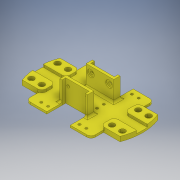
# Autodesk Inventor part: yellow_part-july21
Saved by Autodesk Inventor 2017 SP1 (Build 210196100, 196)
## iProperties
Created: 2016-07-25
Part Number: yellow_part-july21
Material: Verre
Document SubType Name: Modeling
Designer: tmonglon
Density: 2.18 g/cm^3
Appearance: Jaune canari
Mass: 28.4543 g
Surface Area: 129.801 cm^2
Volume: 13.0524 cm^3
Author: tmonglon
Autodesk Inventor part; units mm, degrees
(part 1 of 2)
ref_plane "YZ Plane" through (0, 0, 0) normal (1, 0, 0) x (0, 1, 0)
ref_plane "XZ Plane" through (0, 0, 0) normal (0, 1, 0) x (-1, 0, 0)
ref_plane "XY Plane" through (0, 0, 0) normal (0, 0, 1) x (1, 0, 0)
sketch "Esquisse1" plane through (0, 0, 0) normal (0, 0, 1) x (1, 0, 0)
  line L0 (-50, 42) -> (-50, 18)
  line L1 (-100, 30) -> (0, 30)
  line L2 (-61, 42) -> (-39, 42)
  line L3 (-77, 60) -> (-61.2, 60)
  line L4 (-38.8, 60) -> (-23, 60)
  line L5 (-81, 56) -> (-81, 47.873)
  line L6 (-19, 56) -> (-19, 47.873)
  line L7 (-81, 48) -> (-96.6476, 48)
  line L8 (-19, 48) -> (-3.3524, 48)
  line L9 (-96, 45) -> (-91, 45)
  line L10 (-91, 45) -> (-91, 40)
  line L11 (-91, 40) -> (-96, 40)
  line L12 (-96, 40) -> (-96, 45)
  line L13 (-91, 44) -> (-94, 44)
  line L14 (-94, 44) -> (-94, 41)
  line L15 (-94, 41) -> (-91, 41)
  line L16 (-91, 41) -> (-91, 44)
  line L17 (-86, 45) -> (-81, 45)
  line L18 (-81, 45) -> (-81, 40)
  line L19 (-81, 40) -> (-86, 40)
  line L20 (-86, 40) -> (-86, 45)
  line L21 (-4, 45) -> (-9, 45)
  line L22 (-9, 45) -> (-9, 40)
  line L23 (-9, 40) -> (-4, 40)
  line L24 (-4, 40) -> (-4, 45)
  line L25 (-9, 44) -> (-6, 44)
  line L26 (-6, 44) -> (-6, 41)
  line L27 (-6, 41) -> (-9, 41)
  line L28 (-9, 41) -> (-9, 44)
  line L29 (-14, 45) -> (-19, 45)
  line L30 (-19, 45) -> (-19, 40)
  line L31 (-19, 40) -> (-14, 40)
  line L32 (-14, 40) -> (-14, 45)
  line L33 (-96, 15) -> (-91, 15)
  line L34 (-91, 15) -> (-91, 20)
  line L35 (-91, 20) -> (-96, 20)
  line L36 (-96, 20) -> (-96, 15)
  line L37 (-91, 16) -> (-94, 16)
  line L38 (-94, 16) -> (-94, 19)
  line L39 (-94, 19) -> (-91, 19)
  line L40 (-91, 19) -> (-91, 16)
  line L41 (-86, 15) -> (-81, 15)
  line L42 (-81, 15) -> (-81, 20)
  line L43 (-81, 20) -> (-86, 20)
  line L44 (-86, 20) -> (-86, 15)
  line L45 (-19, 15) -> (-19, 20)
  line L46 (-14, 15) -> (-19, 15)
  line L47 (-14, 20) -> (-14, 15)
  line L48 (-19, 20) -> (-14, 20)
  line L49 (-9, 16) -> (-6, 16)
  line L50 (-6, 19) -> (-9, 19)
  line L51 (-6, 16) -> (-6, 19)
  line L52 (-4, 15) -> (-9, 15)
  line L53 (-4, 20) -> (-4, 15)
  line L54 (-9, 20) -> (-4, 20)
  line L55 (-9, 19) -> (-9, 16)
  line L56 (-9, 15) -> (-9, 20)
  line L57 (-61, 18) -> (-39, 18)
  line L58 (-77, 0) -> (-61.2, 0)
  line L59 (-38.8, 0) -> (-23, 0)
  line L60 (-81, 4) -> (-81, 12.127)
  line L61 (-19, 4) -> (-19, 12.127)
  line L62 (-81, 12) -> (-96.6476, 12)
  line L63 (-19, 12) -> (-3.3524, 12)
  arc A0 (-96.6476, 48) -> (-96.6476, 12) centre (-50, 30) ccw
  arc A1 (-3.3524, 12) -> (-3.3524, 48) centre (-50, 30) ccw
  arc A2 (-96.6476, 48) -> (-96.6476, 12) centre (-50, 30) ccw
  arc A3 (-3.3524, 12) -> (-3.3524, 48) centre (-50, 30) ccw
  line L64 (-23, 0) -> (-38.8, 0)
  line L65 (-61.2, 0) -> (-77, 0)
  line L66 (-78, 44) -> (-78, 39)
  line L67 (-82, 35) -> (-98.5, 35)
  line L68 (-81, 48) -> (-82, 48)
  arc A4 (-82, 35) -> (-78, 39) centre (-82, 39) ccw
  arc A5 (-78, 44) -> (-82, 48) centre (-82, 44) ccw
  arc A6 (-99.707, 35.4053) -> (-98.5, 35) centre (-98.5, 37) ccw
  line L69 (-22, 44) -> (-22, 39)
  line L70 (-18, 35) -> (-1.5, 35)
  arc A7 (-22, 39) -> (-18, 35) centre (-18, 39) ccw
  arc A8 (-18, 48) -> (-22, 44) centre (-18, 44) ccw
  arc A9 (-1.5, 35) -> (-0.293, 35.4053) centre (-1.5, 37) ccw
  line L71 (-78, 16) -> (-78, 21)
  line L72 (-82, 25) -> (-98.5, 25)
  arc A10 (-78, 21) -> (-82, 25) centre (-82, 21) ccw
  arc A11 (-82, 12) -> (-78, 16) centre (-82, 16) ccw
  arc A12 (-98.5, 25) -> (-99.707, 24.5947) centre (-98.5, 23) ccw
  arc A13 (-22, 16) -> (-18, 12) centre (-18, 16) ccw
  line L73 (-22, 16) -> (-22, 21)
  arc A14 (-18, 25) -> (-22, 21) centre (-18, 21) ccw
  line L74 (-18, 25) -> (-1.5, 25)
  arc A15 (-0.293, 24.5947) -> (-1.5, 25) centre (-1.5, 23) ccw
  arc A16 (-77, 60) -> (-81, 56) centre (-77, 56) ccw
  arc A17 (-19, 56) -> (-23, 60) centre (-23, 56) ccw
  arc A18 (-81, 4) -> (-77, 0) centre (-77, 4) ccw
  arc A19 (-23, 0) -> (-19, 4) centre (-23, 4) ccw
  circle A20 centre (-60, 26.75) radius 1
  circle A21 centre (-40, 26.75) radius 1
  circle A22 centre (-40, 33.25) radius 1
  circle A23 centre (-60, 33.25) radius 1
  line L75 (-61, 18) -> (-61.2, 18)
  line L76 (-61.2, 18) -> (-61.2, 0)
  line L77 (-39, 18) -> (-38.8, 18)
  line L78 (-38.8, 18) -> (-38.8, 0)
  line L79 (-61, 42) -> (-61.2, 42)
  line L80 (-61.2, 42) -> (-61.2, 60)
  line L81 (-39, 42) -> (-38.8, 42)
  line L82 (-38.8, 42) -> (-38.8, 60)
  circle A24 centre (-71.5, 55) radius 1
  circle A25 centre (-65, 55) radius 1
  circle A26 centre (-28.5, 55) radius 1
  circle A27 centre (-35, 55) radius 1
  circle A28 centre (-71.5, 5) radius 1
  circle A29 centre (-65, 5) radius 1
  circle A30 centre (-35, 5) radius 1
  circle A31 centre (-28.5, 5) radius 1
  point P0 (0, 0)
  point P1 (-100, 48)
  point P2 (0, 48)
  point P3 (-81, 60)
  point P4 (-19, 60)
  point P5 (-81, 0)
  point P6 (-19, 0)
  dimension "d4" = 22
  dimension "d9" = 5
  dimension "d10" = 5
  dimension "d11" = 3
  dimension "d12" = 3
  dimension "d13" = 1
  dimension "d14" = 10
  dimension "d16" = 5
  dimension "d17" = 5
  dimension "d18" = 5
  dimension "d19" = 22
  dimension "d20" = 13
  dimension "d21" = 4
  dimension "d23" = 4
  dimension "d24" = 1.5
  dimension "d25" = 4
  dimension "d26" = 2
  dimension "d27" = 2
  dimension "d28" = 2
  dimension "d29" = 2
  dimension "d30" = 10
  dimension "d31" = 10
  dimension "d32" = 10
  dimension "d33" = 10
  dimension "d34" = 3.25
  dimension "d35" = 3.25
  dimension "d36" = 3.25
  dimension "d37" = 3.25
  dimension "d42" = 22.4
  dimension "d43" = 22.4
  dimension "d44" = 2
  dimension "d45" = 2
  dimension "d46" = 6.5
  dimension "d47" = 28.5
  dimension "d48" = 5
  constraints: 166 end point, 75 symmetric about line, 50 point on circle, 32 centre point, 24 point on line, 13 tangent, 11 horizontal, 10 parallel, 8 perpendicular, 4 equal radius, 3 midpoint, 2 vertical, 15 other
  measures "d4" distance of L2.start L2.end
  measures "d9" distance of L10.end L11.end
  measures "d10" distance of L9.end L10.end
  measures "d11" distance of L13.start L13.end
  measures "d12" distance of L13.end L14.end
  measures "d13" distance between parallel lines of L9 L13
  measures "d14" distance between parallel lines of L1 L11
  measures "d16" distance of L17.start L17.end
  measures "d17" distance of L17.end L18.end
  measures "d18" distance between parallel lines of L20 L16
  measures "d19" distance from line of L66 L1.start
  measures "d20" distance between parallel lines of L67 L7
  measures "d21" radius of A4
  measures "d23" diameter of A6
  measures "d24" horizontal distance of L1.start A6.centre
  measures "d25" radius of A16
  measures "d26" diameter of A20
  measures "d27" diameter of A21
  measures "d28" diameter of A22
  measures "d29" diameter of A23
  measures "d30" distance from line of L0 A23.centre
  measures "d31" distance from line of L0 A22.centre
  measures "d32" distance from line of L0 A20.centre
  measures "d33" distance from line of A21.centre L0
  measures "d34" distance from line of L1 A23.centre
  measures "d35" distance from line of L1 A20.centre
  measures "d36" distance from line of L1 A21.centre
  measures "d37" distance from line of L1 A22.centre
  measures "d42" distance between parallel lines of L82 L80
  measures "d43" distance between parallel lines of L78 L76
  measures "d44" diameter of A24
  measures "d45" diameter of A25
  measures "d46" distance of A25.centre A24.centre
  measures "d47" horizontal distance of L1.start A24.centre
  measures "d48" distance from line of L3 A24.centre
extrude "Extrusion1" add sketch "Esquisse1" against normal blind 2 contours L2 L81 L82 L4 A17 L6 A8 L69 A7 L70 A9 A1 L1 L0 | L0 L1 A0 A6 L67 A4 L66 A5 L5 A16 L3 L80 L79 L2 | L1 A1 A15 L74 A14 L73 A13 L61 A19 L59 L78 L77 L57 L0 | L0 L57 L75 L76 L58 A18 L60 A11 L71 A10 L72 A12 A0 L1 | A0 L7 A5 L66 A4 L67 A6 | A12 L72 A10 L71 A11 L62 A0 | A1 L63 A13 L73 A14 L74 A15 | A9 L70 A7 L69 A8 L8 A1 | L7 L5 A5 | A11 L60 L62 | L63 L61 A13 | A8 L6 L8 | L9 L10 L13 L14 L15 L11 L12 | L24 L23 L22 L27 L26 L25 L21 | L36 L35 L34 L39 L38 L37 L33 | L49 L51 L50 L56 L54 L53 L52
extrude "Extrusion3" add sketch "Esquisse1" along normal blind 2.5 contours A0 L7 A5 L66 A4 L67 A6 | L9 L10 L13 L14 L15 L11 L12
extrude "Extrusion4" add sketch "Esquisse1" along normal blind 2.5 contours A1 L63 A13 L73 A14 L74 A15 | L49 L51 L50 L56 L54 L53 L52
sketch "Esquisse4" plane through (0, 0, 0) normal (0, 0, 1) x (1, 0, 0)
  line L0 (-91, 44) -> (-91, 41) projected
  line L1 (-91, 41) -> (-94, 41) projected
  line L2 (-94, 41) -> (-94, 44) projected
  line L3 (-94, 44) -> (-91, 44) projected
  arc A0 (-78, 44) -> (-82, 48) centre (-82, 44) ccw projected
  line L4 (-82, 48) -> (-96.6476, 48) projected
  arc A1 (-96.6476, 48) -> (-99.707, 35.4053) centre (-50, 30) ccw projected
  arc A2 (-99.707, 35.4053) -> (-98.5, 35) centre (-98.5, 37) ccw projected
  line L5 (-98.5, 35) -> (-82, 35) projected
  arc A3 (-82, 35) -> (-78, 39) centre (-82, 39) ccw projected
  line L6 (-78, 39) -> (-78, 44) projected
  line L7 (-81, 45) -> (-81, 40) projected
  line L8 (-81, 40) -> (-86, 40) projected
  line L9 (-86, 40) -> (-86, 45) projected
  line L10 (-86, 45) -> (-81, 45) projected
  line L11 (-9, 16) -> (-9, 19) projected
  line L12 (-9, 19) -> (-6, 19) projected
  line L13 (-6, 19) -> (-6, 16) projected
  line L14 (-6, 16) -> (-9, 16) projected
  line L15 (-19, 15) -> (-19, 20) projected
  line L16 (-19, 20) -> (-14, 20) projected
  line L17 (-14, 20) -> (-14, 15) projected
  line L18 (-14, 15) -> (-19, 15) projected
  arc A4 (-3.3524, 12) -> (-0.293, 24.5947) centre (-50, 30) ccw projected
  arc A5 (-0.293, 24.5947) -> (-1.5, 25) centre (-1.5, 23) ccw projected
  line L19 (-1.5, 25) -> (-18, 25) projected
  arc A6 (-18, 25) -> (-22, 21) centre (-18, 21) ccw projected
  line L20 (-22, 21) -> (-22, 16) projected
  arc A7 (-22, 16) -> (-18, 12) centre (-18, 16) ccw projected
  line L21 (-18, 12) -> (-3.3524, 12) projected
  line L22 (-50, 30) -> (-66.4619, 30)
  line L23 (-91, 16) -> (-91, 19)
  line L24 (-91, 19) -> (-94, 19)
  line L25 (-94, 19) -> (-94, 16)
  line L26 (-94, 16) -> (-91, 16)
  arc A8 (-82, 12) -> (-78, 16) centre (-82, 16) ccw
  line L27 (-82, 12) -> (-96.6476, 12)
  arc A9 (-99.707, 24.5947) -> (-96.6476, 12) centre (-50, 30) ccw
  arc A10 (-98.5, 25) -> (-99.707, 24.5947) centre (-98.5, 23) ccw
  line L28 (-98.5, 25) -> (-82, 25)
  arc A11 (-78, 21) -> (-82, 25) centre (-82, 21) ccw
  line L29 (-78, 21) -> (-78, 16)
  line L30 (-81, 15) -> (-81, 20)
  line L31 (-81, 20) -> (-86, 20)
  line L32 (-86, 20) -> (-86, 15)
  line L33 (-86, 15) -> (-81, 15)
  line L34 (-9, 44) -> (-9, 41)
  line L35 (-9, 41) -> (-6, 41)
  line L36 (-6, 41) -> (-6, 44)
  line L37 (-6, 44) -> (-9, 44)
  line L38 (-19, 45) -> (-19, 40)
  line L39 (-19, 40) -> (-14, 40)
  line L40 (-14, 40) -> (-14, 45)
  line L41 (-14, 45) -> (-19, 45)
  arc A12 (-0.293, 35.4053) -> (-3.3524, 48) centre (-50, 30) ccw
  arc A13 (-1.5, 35) -> (-0.293, 35.4053) centre (-1.5, 37) ccw
  line L42 (-1.5, 35) -> (-18, 35)
  arc A14 (-22, 39) -> (-18, 35) centre (-18, 39) ccw
  line L43 (-22, 39) -> (-22, 44)
  arc A15 (-18, 48) -> (-22, 44) centre (-18, 44) ccw
  line L44 (-18, 48) -> (-3.3524, 48)
  point P0 (0, 0)
  constraints: 46 end point, 36 symmetric about line, 16 point on circle, 8 centre point, 1 horizontal, 8 other
extrude "Extrusion5" add sketch "Esquisse4" along normal blind 2.5 contours L27 A9 A10 L28 A11 L29 A8 | A13 L42 A14 L43 A15 L44 A12
sketch "Esquisse6" plane through (0, 0, 2.5) normal (0, 0, 1) x (1, 0, 0)
  arc A0 (-98.5, 25) -> (-99.707, 24.5947) centre (-98.5, 23) ccw projected
  line L0 (-98.5, 25) -> (-82, 25) projected
  arc A1 (-78, 21) -> (-82, 25) centre (-82, 21) ccw projected
  line L1 (-78, 21) -> (-78, 16) projected
  arc A2 (-82, 12) -> (-78, 16) centre (-82, 16) ccw projected
  line L2 (-82, 12) -> (-96.6476, 12) projected
  arc A3 (-99.707, 24.5947) -> (-96.6476, 12) centre (-50, 30) ccw projected
  arc A4 (-1.5, 35) -> (-0.293, 35.4053) centre (-1.5, 37) ccw projected
  line L3 (-1.5, 35) -> (-18, 35) projected
  arc A5 (-22, 39) -> (-18, 35) centre (-18, 39) ccw projected
  line L4 (-22, 39) -> (-22, 44) projected
  arc A6 (-18, 48) -> (-22, 44) centre (-18, 44) ccw projected
  line L5 (-18, 48) -> (-3.3524, 48) projected
  arc A7 (-0.293, 35.4053) -> (-3.3524, 48) centre (-50, 30) ccw projected
  arc A8 (-22, 16) -> (-18, 12) centre (-18, 16) ccw projected
  line L6 (-22, 16) -> (-22, 21) projected
  arc A9 (-18, 25) -> (-22, 21) centre (-18, 21) ccw projected
  line L7 (-18, 25) -> (-1.5, 25) projected
  arc A10 (-0.293, 24.5947) -> (-1.5, 25) centre (-1.5, 23) ccw projected
  arc A11 (-3.3524, 12) -> (-0.293, 24.5947) centre (-50, 30) ccw projected
  line L8 (-3.3524, 12) -> (-18, 12) projected
  arc A12 (-99.707, 35.4053) -> (-98.5, 35) centre (-98.5, 37) ccw projected
  arc A13 (-96.6476, 48) -> (-99.707, 35.4053) centre (-50, 30) ccw projected
  line L9 (-96.6476, 48) -> (-82, 48) projected
  arc A14 (-78, 44) -> (-82, 48) centre (-82, 44) ccw projected
  line L10 (-78, 44) -> (-78, 39) projected
  arc A15 (-82, 35) -> (-78, 39) centre (-82, 39) ccw projected
  line L11 (-82, 35) -> (-98.5, 35) projected
  line L12 (-14, 15) -> (-14, 20) projected
  line L13 (-14, 20) -> (-19, 20) projected
  line L14 (-19, 20) -> (-19, 15) projected
  line L15 (-19, 15) -> (-14, 15) projected
  line L16 (-86, 45) -> (-86, 40) projected
  line L17 (-86, 40) -> (-81, 40) projected
  line L18 (-81, 40) -> (-81, 45) projected
  line L19 (-81, 45) -> (-86, 45) projected
  line L20 (-81, 20) -> (-86, 20) projected
  line L21 (-86, 20) -> (-86, 15) projected
  line L22 (-86, 15) -> (-81, 15) projected
  line L23 (-81, 15) -> (-81, 20) projected
  line L24 (-9, 41) -> (-6, 41) projected
  line L25 (-6, 41) -> (-6, 44) projected
  line L26 (-6, 44) -> (-9, 44) projected
  line L27 (-9, 44) -> (-9, 41) projected
  line L28 (-19, 45) -> (-19, 40) projected
  line L29 (-19, 40) -> (-14, 40) projected
  line L30 (-14, 40) -> (-14, 45) projected
  line L31 (-14, 45) -> (-19, 45) projected
  line L32 (-94, 44) -> (-94, 41) projected
  line L33 (-94, 41) -> (-91, 41) projected
  line L34 (-91, 41) -> (-91, 44) projected
  line L35 (-91, 44) -> (-94, 44) projected
  line L36 (-6, 16) -> (-6, 19) projected
  line L37 (-6, 19) -> (-9, 19) projected
  line L38 (-9, 19) -> (-9, 16) projected
  line L39 (-9, 16) -> (-6, 16) projected
  line L40 (-91, 19) -> (-94, 19) projected
  line L41 (-94, 19) -> (-94, 16) projected
  line L42 (-94, 16) -> (-91, 16) projected
  line L43 (-91, 16) -> (-91, 19) projected
  line L44 (-91, 45) -> (-96, 45)
  line L45 (-96, 45) -> (-96, 40)
  line L46 (-96, 40) -> (-91, 40)
  line L47 (-91, 40) -> (-91, 45)
  line L48 (-91, 44) -> (-91, 41) projected
  line L49 (-91, 20) -> (-96, 20)
  line L50 (-96, 20) -> (-96, 15)
  line L51 (-96, 15) -> (-91, 15)
  line L52 (-91, 15) -> (-91, 20)
  line L53 (-50, 30) -> (-50, 35)
  line L54 (-6, 44) -> (-6, 41)
  line L55 (-6, 41) -> (-9, 41)
  line L56 (-9, 41) -> (-9, 44)
  line L57 (-9, 44) -> (-6, 44)
  line L58 (-9, 19) -> (-6, 19)
  line L59 (-6, 19) -> (-6, 16)
  line L60 (-6, 16) -> (-9, 16)
  line L61 (-9, 16) -> (-9, 19)
  line L62 (-9, 45) -> (-4, 45)
  line L63 (-4, 45) -> (-4, 40)
  line L64 (-4, 40) -> (-9, 40)
  line L65 (-9, 40) -> (-9, 45)
  line L66 (-9, 44) -> (-9, 41)
  line L67 (-9, 20) -> (-4, 20)
  line L68 (-4, 20) -> (-4, 15)
  line L69 (-4, 15) -> (-9, 15)
  line L70 (-9, 15) -> (-9, 20)
  point P0 (0, 0)
  dimension "d59" = 5
  dimension "d60" = 5
  dimension "d61" = 1
  dimension "d62" = 5
  dimension "d63" = 5
  dimension "d64" = 1
  constraints: 52 end point, 8 symmetric about line, 4 parallel, 2 horizontal, 2 perpendicular, 1 collinear, 1 vertical
  measures "d59" distance of L44.end L45.end
  measures "d60" distance of L45.end L46.end
  measures "d61" distance between parallel lines of L46 L33
  measures "d62" distance of L49.end L50.end
  measures "d63" distance of L49.start L49.end
  measures "d64" distance between parallel lines of L51 L42
extrude "Extrusion6" cut sketch "Esquisse6" against normal blind 3 contours L27 L26 L25 L24 | L24 L25 L26 L65 L62 L63 L64 | L35 L34 L33 L32 | L32 L33 L47 L46 L45 L44 L35 | L36 L37 L70 L67 L68 L69 L39 | L43 L42 L41 L40 | L40 L41 L42 L52 L51 L50 L49
sketch "Esquisse7" plane through (0, 0, -2) normal (0, 0, -1) x (-1, 0, 0)
  line L0 (91, 44) -> (94, 44) projected
  line L1 (94, 44) -> (94, 41) projected
  line L2 (94, 41) -> (91, 41) projected
  line L3 (91, 41) -> (91, 44) projected
  line L4 (86, 45) -> (86, 40) projected
  line L5 (86, 40) -> (81, 40) projected
  line L6 (81, 40) -> (81, 45) projected
  line L7 (81, 45) -> (86, 45) projected
  line L8 (91, 19) -> (94, 19) projected
  line L9 (94, 19) -> (94, 16) projected
  line L10 (94, 16) -> (91, 16) projected
  line L11 (91, 16) -> (91, 19) projected
  line L12 (81, 20) -> (86, 20) projected
  line L13 (86, 20) -> (86, 15) projected
  line L14 (86, 15) -> (81, 15) projected
  line L15 (81, 15) -> (81, 20) projected
  circle A0 centre (65, 5) radius 1 projected
  circle A1 centre (71.5, 5) radius 1 projected
  circle A2 centre (60, 26.75) radius 1 projected
  arc A3 (96.6476, 12) -> (96.6476, 48) centre (50, 30) ccw projected
  line L16 (96.6476, 48) -> (81, 48) projected
  line L17 (81, 48) -> (81, 56) projected
  arc A4 (81, 56) -> (77, 60) centre (77, 56) ccw projected
  line L18 (77, 60) -> (61.2, 60) projected
  line L19 (61.2, 60) -> (61.2, 42) projected
  line L20 (61.2, 42) -> (38.8, 42) projected
  line L21 (38.8, 42) -> (38.8, 60) projected
  line L22 (38.8, 60) -> (23, 60) projected
  arc A5 (23, 60) -> (19, 56) centre (23, 56) ccw projected
  line L23 (19, 56) -> (19, 48) projected
  line L24 (19, 48) -> (3.3524, 48) projected
  arc A6 (3.3524, 48) -> (3.3524, 12) centre (50, 30) ccw projected
  line L25 (3.3524, 12) -> (19, 12) projected
  line L26 (19, 12) -> (19, 4) projected
  arc A7 (19, 4) -> (23, 0) centre (23, 4) ccw projected
  line L27 (23, 0) -> (38.8, 0) projected
  line L28 (38.8, 0) -> (38.8, 18) projected
  line L29 (38.8, 18) -> (61.2, 18) projected
  line L30 (61.2, 18) -> (61.2, 0) projected
  line L31 (61.2, 0) -> (77, 0) projected
  arc A8 (77, 0) -> (81, 4) centre (77, 4) ccw projected
  line L32 (81, 4) -> (81, 12) projected
  line L33 (81, 12) -> (96.6476, 12) projected
  circle A9 centre (40, 33.25) radius 1 projected
  circle A10 centre (35, 55) radius 1 projected
  circle A11 centre (28.5, 55) radius 1 projected
  line L34 (19, 45) -> (19, 40) projected
  line L35 (19, 40) -> (14, 40) projected
  line L36 (14, 40) -> (14, 45) projected
  line L37 (14, 45) -> (19, 45) projected
  line L38 (9, 41) -> (6, 41) projected
  line L39 (6, 41) -> (6, 44) projected
  line L40 (6, 44) -> (9, 44) projected
  line L41 (9, 44) -> (9, 41) projected
  line L42 (14, 15) -> (14, 20) projected
  line L43 (14, 20) -> (19, 20) projected
  line L44 (19, 20) -> (19, 15) projected
  line L45 (19, 15) -> (14, 15) projected
  circle A12 centre (35, 5) radius 1 projected
  circle A13 centre (28.5, 5) radius 1 projected
  circle A14 centre (40, 26.75) radius 1 projected
  circle A15 centre (65, 55) radius 1 projected
  circle A16 centre (71.5, 55) radius 1 projected
  circle A17 centre (60, 33.25) radius 1 projected
  line L46 (9, 16) -> (6, 16) projected
  line L47 (6, 16) -> (6, 19) projected
  line L48 (6, 19) -> (9, 19) projected
  line L49 (9, 19) -> (9, 16) projected
  line L50 (61.2, 18) -> (38.8, 18)
  line L51 (38, 20.5) -> (62, 20.5)
  line L52 (61.2, 42) -> (38.8, 42)
  line L53 (38, 39.5) -> (62, 39.5)
  line L54 (61.2, 42) -> (38.8, 42) projected
  line L55 (38.8, 20.5) -> (36.8, 20.5)
  line L56 (36.8, 20.5) -> (36.8, 14.5)
  line L57 (36.8, 14.5) -> (38.8, 14.5)
  line L58 (38.8, 14.5) -> (38.8, 18)
  line L59 (38.8, 0) -> (38.8, 18) projected
  line L60 (38.8, 39.5) -> (36.8, 39.5)
  line L61 (36.8, 39.5) -> (36.8, 45.5)
  line L62 (36.8, 45.5) -> (38.8, 45.5)
  line L63 (38.8, 45.5) -> (38.8, 42)
  line L64 (61.1821, 39.5) -> (63.1821, 39.5)
  line L65 (63.1821, 39.5) -> (63.1821, 45.5)
  line L66 (63.1821, 45.5) -> (61.1821, 45.5)
  line L67 (61.1821, 45.5) -> (61.1821, 42)
  line L68 (61.1821, 20.5) -> (63.1821, 20.5)
  line L69 (63.1821, 20.5) -> (63.1821, 14.5)
  line L70 (63.1821, 14.5) -> (61.1821, 14.5)
  line L71 (61.1821, 14.5) -> (61.1821, 18)
  point P0 (0, 0)
  dimension "d70" = 22.4
  dimension "d72" = 6
  dimension "d73" = 2
  dimension "d74" = 2
  dimension "d75" = 6
  dimension "d76" = 2
  dimension "d77" = 6
  dimension "d78" = 2
  constraints: 40 end point, 13 point on line, 10 parallel, 6 horizontal, 4 perpendicular, 2 collinear
  measures "d70" distance between parallel lines of L30 L28
  measures "d72" distance of L55.end L56.end
  measures "d73" distance of L56.end L57.end
  measures "d74" distance of L61.end L62.end
  measures "d75" distance of L60.end L61.end
  measures "d76" distance of L65.end L66.end
  measures "d77" distance of L68.end L69.end
  measures "d78" distance of L69.end L70.end
extrude "Extrusion7" add sketch "Esquisse7" against normal blind 21 contours L70 L71 L29 L30 | L30 L29 L28 L57 L56 L55 L51 L68 L69 L70 | L66 L65 L64 L53 L60 L61 L62 L21 L20 L19 | L19 L20 L67 L66
sketch "Esquisse8" plane through (-61.1821, 18, -2) normal (0, -1, 0) x (1, 0, 0)
  line L0 (0, 21) -> (0, 0) projected
  line L1 (22.3821, 0) -> (0, 0) projected
  line L2 (22.3821, 0) -> (22.3821, 21) projected
  line L3 (0, 21) -> (22.3821, 21) projected
  line L4 (-2, 21) -> (24.3821, 21) projected
  line L5 (11.1911, 21) -> (11.1911, 2)
  line L6 (-2, 2) -> (24.3821, 2) projected
  circle A0 centre (2.4411, 15.2) radius 1.25
  circle A1 centre (19.9411, 15.2) radius 1.25
  point P0 (61.1821, 2)
  dimension "d81" = 2.5
  dimension "d82" = 5.8
  dimension "d83" = 8.75
  constraints: 2 centre point, 2 end point, 2 midpoint, 1 symmetric about line, 1 other
  measures "d81" diameter of A0
  measures "d82" distance from line of L3 A0.centre
  measures "d83" distance from line of L5 A0.centre
extrude "Extrusion8" cut sketch "Esquisse8" against normal through all contours A0 | A1
hole "Perçage1" at (-58.7411, 39.5, 13.2) direction (0, 1, 0) diameter 6.6 depth 1
hole "Perçage2" at (-41.2411, 39.5, 13.2) direction (0, 1, 0) diameter 6.6 depth 1
hole "Perçage3" at (-41.2411, 20.5, 13.2) direction (0, -1, 0) diameter 6.6 depth 1
hole "Perçage4" at (-58.7411, 20.5, 13.2) direction (0, -1, 0) diameter 6.6 depth 1
fillet "Congé1" radius 2 2 edges at (-49.9911, 20.5, 0) (-49.9911, 39.5, 0)
fillet "Congé2" radius 2 8 edges at (-36.8, 21.5, 0) (-36.8, 17.5, 0) (-36.8, 42.5, 0) (-36.8, 38.5, 0) (-63.1821, 21.5, 0) (-63.1821, 17.5, 0) (-63.1821, 42.5, 0) (-63.1821, 38.5, 0)
fillet "Congé3" radius 2 8 edges at (-35.8, 14.5, 0) (-37.8, 14.5, 0) (-64.1821, 14.5, 0) (-62.1911, 14.5, 0) (-62.1911, 45.5, 0) (-64.1821, 45.5, 0) (-37.8, 45.5, 0) (-35.8, 45.5, 0)
sketch "Esquisse9" plane through (0, 0, -2) normal (0, 0, -1) x (-1, 0, 0)
  line L0 (20.3471, 14.8582) -> (37.5767, 14.8582) construction
  line L1 (37.5767, 14.8582) -> (37.5767, 7.8153) construction
  line L2 (37.5767, 7.8153) -> (20.3471, 7.8153) construction
  line L3 (20.3471, 7.8153) -> (20.3471, 14.8582) construction
  line L4 (66.5479, 9.4629) -> (66.5479, 31.182) construction
  line L5 (66.5479, 31.182) -> (77.9246, 31.182) construction
  line L6 (77.9246, 31.182) -> (77.9246, 9.4629) construction
  line L7 (77.9246, 9.4629) -> (66.5479, 9.4629) construction
  line L8 (25.3892, 14.7346) -> (23.2883, 8.6346)
  line L9 (23.2883, 8.6346) -> (22.4134, 8.6346)
  line L10 (22.4134, 8.6346) -> (20.3125, 14.7346)
  line L11 (20.3125, 14.7346) -> (21.1825, 14.7346)
  line L12 (21.1825, 14.7346) -> (22.8731, 9.6677)
  line L13 (22.8731, 9.6677) -> (24.5637, 14.7346)
  line L14 (24.5637, 14.7346) -> (25.3892, 14.7346)
  line L15 (29.2548, 8.6346) -> (26.279, 8.6346)
  line L16 (26.279, 8.6346) -> (26.279, 9.2574)
  line L17 (26.279, 9.2574) -> (27.3863, 9.2574)
  line L18 (27.3863, 9.2574) -> (27.3863, 13.3455)
  line L19 (27.3863, 13.3455) -> (26.279, 13.3455)
  line L20 (26.279, 13.3455) -> (26.279, 13.9041)
  spline S0 degree 2 poles (26.279, 13.9041) (26.9068, 13.9041) (27.5, 14.26) (27.5395, 14.7544) knots 0 0 0 1 2 2 2
  line L21 (27.5395, 14.7544) -> (28.1723, 14.7544)
  line L22 (28.1723, 14.7544) -> (28.1723, 9.2574)
  line L23 (28.1723, 9.2574) -> (29.2548, 9.2574)
  line L24 (29.2548, 9.2574) -> (29.2548, 8.6346)
  line L25 (31.6869, 8.6346) -> (30.7082, 8.6346)
  line L26 (30.7082, 8.6346) -> (30.7082, 9.8012)
  line L27 (30.7082, 9.8012) -> (31.6869, 9.8012)
  line L28 (31.6869, 9.8012) -> (31.6869, 8.6346)
  spline S1 degree 2 poles (36.7142, 11.6846) (36.7142, 10.0434) (35.7602, 8.5061) (34.7666, 8.5061) knots 0 0 0 1 2 2 2
  spline S2 degree 2 poles (34.7666, 8.5061) (33.7582, 8.5061) (32.814, 10.0731) (32.814, 11.6796) knots 0 0 0 1 2 2 2
  spline S3 degree 2 poles (32.814, 11.6796) (32.814, 13.3307) (33.7681, 14.8582) (34.7666, 14.8582) knots 0 0 0 1 2 2 2
  spline S4 degree 2 poles (34.7666, 14.8582) (35.7701, 14.8582) (36.7142, 13.2763) (36.7142, 11.6846) knots 0 0 0 1 2 2 2
  spline S5 degree 2 poles (35.6663, 9.8259) (35.7849, 10.1275) (35.8838, 11.0568) (35.8838, 11.6846) knots 0 0 0 1 2 2 2
  spline S6 degree 2 poles (35.8838, 11.6846) (35.8838, 12.3124) (35.7849, 13.2368) (35.6613, 13.5482) knots 0 0 0 1 2 2 2
  spline S7 degree 2 poles (35.6613, 13.5482) (35.5377, 13.8596) (35.1077, 14.1809) (34.7666, 14.1809) knots 0 0 0 1 2 2 2
  spline S8 degree 2 poles (34.7666, 14.1809) (34.4255, 14.1809) (33.9856, 13.8596) (33.857, 13.5383) knots 0 0 0 1 2 2 2
  spline S9 degree 2 poles (33.857, 13.5383) (33.7335, 13.2269) (33.6445, 12.2778) (33.6445, 11.6796) knots 0 0 0 1 2 2 2
  spline S10 degree 2 poles (33.6445, 11.6796) (33.6445, 11.037) (33.7236, 10.1769) (33.8521, 9.8407) knots 0 0 0 1 2 2 2
  spline S11 degree 2 poles (33.8521, 9.8407) (33.9707, 9.5244) (34.4107, 9.1833) (34.7666, 9.1833) knots 0 0 0 1 2 2 2
  spline S12 degree 2 poles (34.7666, 9.1833) (35.1027, 9.1833) (35.5427, 9.5046) (35.6663, 9.8259) knots 0 0 0 1 2 2 2
  line L29 (70.2039, 12.3587) -> (70.2039, 11.8936)
  line L30 (70.2039, 11.8936) -> (68.4908, 11.8936)
  line L31 (68.4908, 11.8936) -> (68.4908, 10.2826)
  line L32 (68.4908, 10.2826) -> (70.2039, 10.2826)
  line L33 (70.2039, 10.2826) -> (70.2039, 9.8174)
  line L34 (70.2039, 9.8174) -> (66.7039, 9.8174)
  line L35 (66.7039, 9.8174) -> (66.7039, 10.2826)
  line L36 (66.7039, 10.2826) -> (68.0767, 10.2826)
  line L37 (68.0767, 10.2826) -> (68.0767, 11.8936)
  line L38 (68.0767, 11.8936) -> (66.7039, 11.8936)
  line L39 (66.7039, 11.8936) -> (66.7039, 12.3587)
  line L40 (66.7039, 12.3587) -> (70.2039, 12.3587)
  spline S13 degree 2 poles (70.2635, 14.174) (70.2635, 13.5443) (69.5572, 12.8523) (68.9049, 12.8523) knots 0 0 0 1 2 2 2
  spline S14 degree 2 poles (68.9049, 12.8523) (68.2639, 12.8523) (67.5037, 13.5245) (67.5037, 14.0662) knots 0 0 0 1 2 2 2
  spline S15 degree 2 poles (67.5037, 14.0662) (67.5037, 14.3101) (67.6455, 14.6874) (67.7959, 14.8263) knots 0 0 0 1 2 2 2
  spline S16 degree 2 poles (67.7959, 14.8263) (67.9462, 14.9682) (68.3801, 15.1185) (68.695, 15.1185) knots 0 0 0 1 2 2 2
  line L41 (68.695, 15.1185) -> (68.9361, 15.1185)
  line L42 (68.9361, 15.1185) -> (68.9361, 13.3004)
  spline S17 degree 2 poles (68.9361, 13.3004) (69.3927, 13.3004) (69.8777, 13.7599) (69.8777, 14.1683) knots 0 0 0 1 2 2 2
  spline S18 degree 2 poles (69.8777, 14.1683) (69.8777, 14.313) (69.8125, 14.5938) (69.7614, 14.7072) knots 0 0 0 1 2 2 2
  spline S19 degree 2 poles (69.7614, 14.7072) (69.7047, 14.8263) (69.6054, 14.9908) (69.56, 15.0447) knots 0 0 0 1 2 2 2
  line L43 (69.56, 15.0447) -> (69.56, 15.0703)
  line L44 (69.56, 15.0703) -> (70.0422, 15.0703)
  spline S20 degree 2 poles (70.0422, 15.0703) (70.0734, 14.9937) (70.1642, 14.7611) (70.1897, 14.6703) knots 0 0 0 1 2 2 2
  spline S21 degree 2 poles (70.1897, 14.6703) (70.2266, 14.5427) (70.2635, 14.3328) (70.2635, 14.174) knots 0 0 0 1 2 2 2
  spline S22 degree 2 poles (68.5985, 14.6874) (68.4199, 14.6817) (68.1589, 14.6079) (68.071, 14.537) knots 0 0 0 1 2 2 2
  spline S23 degree 2 poles (68.071, 14.537) (67.9717, 14.4605) (67.8668, 14.2194) (67.8668, 14.0407) knots 0 0 0 1 2 2 2
  spline S24 degree 2 poles (67.8668, 14.0407) (67.8668, 13.8648) (67.9717, 13.6181) (68.0738, 13.516) knots 0 0 0 1 2 2 2
  spline S25 degree 2 poles (68.0738, 13.516) (68.1788, 13.4167) (68.4312, 13.3146) (68.5985, 13.3004) knots 0 0 0 1 2 2 2
  line L45 (68.5985, 13.3004) -> (68.5985, 14.6874)
  line L46 (70.2039, 17.6087) -> (70.2039, 17.1663)
  line L47 (70.2039, 17.1663) -> (69.9146, 17.1663)
  spline S26 degree 2 poles (69.9146, 17.1663) (70.0933, 16.9621) (70.2776, 16.5962) (70.2776, 16.3693) knots 0 0 0 1 2 2 2
  spline S27 degree 2 poles (70.2776, 16.3693) (70.2776, 16.1991) (70.1642, 15.8956) (70.0422, 15.785) knots 0 0 0 1 2 2 2
  spline S28 degree 2 poles (70.0422, 15.785) (69.9203, 15.6716) (69.5487, 15.5468) (69.2821, 15.5468) knots 0 0 0 1 2 2 2
  line L48 (69.2821, 15.5468) -> (67.5775, 15.5468)
  line L49 (67.5775, 15.5468) -> (67.5775, 15.9892)
  line L50 (67.5775, 15.9892) -> (69.075, 15.9892)
  spline S29 degree 2 poles (69.075, 15.9892) (69.2849, 15.9892) (69.56, 16.0204) (69.6622, 16.0743) knots 0 0 0 1 2 2 2
  spline S30 degree 2 poles (69.6622, 16.0743) (69.7643, 16.1282) (69.8579, 16.3126) (69.8579, 16.4856) knots 0 0 0 1 2 2 2
  spline S31 degree 2 poles (69.8579, 16.4856) (69.8579, 16.6472) (69.6735, 17.0131) (69.5402, 17.1663) knots 0 0 0 1 2 2 2
  line L51 (69.5402, 17.1663) -> (67.5775, 17.1663)
  line L52 (67.5775, 17.1663) -> (67.5775, 17.6087)
  line L53 (67.5775, 17.6087) -> (70.2039, 17.6087)
  line L54 (70.2039, 20.2692) -> (70.2039, 19.8267)
  line L55 (70.2039, 19.8267) -> (69.9373, 19.8267)
  spline S32 degree 2 poles (69.9373, 19.8267) (70.0224, 19.7246) (70.1358, 19.5743) (70.184, 19.4722) knots 0 0 0 1 2 2 2
  spline S33 degree 2 poles (70.184, 19.4722) (70.2294, 19.3786) (70.2776, 19.1772) (70.2776, 19.0439) knots 0 0 0 1 2 2 2
  spline S34 degree 2 poles (70.2776, 19.0439) (70.2776, 18.8284) (70.0989, 18.4653) (69.9259, 18.3377) knots 0 0 0 1 2 2 2
  spline S35 degree 2 poles (69.9259, 18.3377) (69.7529, 18.21) (69.2424, 18.0682) (68.9105, 18.0682) knots 0 0 0 1 2 2 2
  spline S36 degree 2 poles (68.9105, 18.0682) (68.5645, 18.0682) (68.0596, 18.2469) (67.8696, 18.4029) knots 0 0 0 1 2 2 2
  spline S37 degree 2 poles (67.8696, 18.4029) (67.6994, 18.5476) (67.5037, 18.9532) (67.5037, 19.1772) knots 0 0 0 1 2 2 2
  spline S38 degree 2 poles (67.5037, 19.1772) (67.5037, 19.3729) (67.5917, 19.6651) (67.6824, 19.8267) knots 0 0 0 1 2 2 2
  line L56 (67.6824, 19.8267) -> (66.5479, 19.8267)
  line L57 (66.5479, 19.8267) -> (66.5479, 20.2692)
  line L58 (66.5479, 20.2692) -> (70.2039, 20.2692)
  line L59 (69.5657, 19.8267) -> (68.0483, 19.8267)
  spline S39 degree 2 poles (68.0483, 19.8267) (67.9689, 19.6622) (67.9093, 19.4013) (67.9093, 19.251) knots 0 0 0 1 2 2 2
  spline S40 degree 2 poles (67.9093, 19.251) (67.9093, 18.9106) (68.4199, 18.5249) (68.902, 18.5249) knots 0 0 0 1 2 2 2
  spline S41 degree 2 poles (68.902, 18.5249) (69.3672, 18.5249) (69.8579, 18.8199) (69.8579, 19.146) knots 0 0 0 1 2 2 2
  spline S42 degree 2 poles (69.8579, 19.146) (69.8579, 19.319) (69.699, 19.6707) (69.5657, 19.8267) knots 0 0 0 1 2 2 2
  line L60 (70.2039, 21.3612) -> (70.2039, 20.9187)
  line L61 (70.2039, 20.9187) -> (67.5775, 20.9187)
  line L62 (67.5775, 20.9187) -> (67.5775, 21.3612)
  line L63 (67.5775, 21.3612) -> (70.2039, 21.3612)
  line L64 (67.1407, 21.3924) -> (67.1407, 20.8904)
  line L65 (67.1407, 20.8904) -> (66.6812, 20.8904)
  line L66 (66.6812, 20.8904) -> (66.6812, 21.3924)
  line L67 (66.6812, 21.3924) -> (67.1407, 21.3924)
  spline S43 degree 2 poles (69.9259, 23.4742) (69.9656, 23.4203) (70.1075, 23.2388) (70.15, 23.1537) knots 0 0 0 1 2 2 2
  spline S44 degree 2 poles (70.15, 23.1537) (70.2124, 23.0374) (70.2776, 22.819) (70.2776, 22.6205) knots 0 0 0 1 2 2 2
  spline S45 degree 2 poles (70.2776, 22.6205) (70.2776, 22.4588) (70.1557, 22.1667) (70.0451, 22.0561) knots 0 0 0 1 2 2 2
  spline S46 degree 2 poles (70.0451, 22.0561) (69.9373, 21.9511) (69.6196, 21.8235) (69.4438, 21.8235) knots 0 0 0 1 2 2 2
  spline S47 degree 2 poles (69.4438, 21.8235) (69.1715, 21.8235) (68.7857, 22.0532) (68.6751, 22.3028) knots 0 0 0 1 2 2 2
  spline S48 degree 2 poles (68.6751, 22.3028) (68.573, 22.5241) (68.4964, 23.1254) (68.4766, 23.4742) knots 0 0 0 1 2 2 2
  line L68 (68.4766, 23.4742) -> (68.3915, 23.4742)
  spline S49 degree 2 poles (68.3915, 23.4742) (68.2383, 23.4742) (68.0483, 23.3806) (67.9944, 23.2955) knots 0 0 0 1 2 2 2
  spline S50 degree 2 poles (67.9944, 23.2955) (67.9405, 23.2105) (67.9065, 22.9665) (67.9065, 22.8361) knots 0 0 0 1 2 2 2
  spline S51 degree 2 poles (67.9065, 22.8361) (67.9065, 22.6829) (67.9972, 22.2688) (68.0852, 22.0617) knots 0 0 0 1 2 2 2
  line L69 (68.0852, 22.0617) -> (68.0852, 22.0362)
  line L70 (68.0852, 22.0362) -> (67.6342, 22.0362)
  spline S52 degree 2 poles (67.6342, 22.0362) (67.6002, 22.1582) (67.5151, 22.6148) (67.5151, 22.8389) knots 0 0 0 1 2 2 2
  spline S53 degree 2 poles (67.5151, 22.8389) (67.5151, 23.1112) (67.6002, 23.4827) (67.7108, 23.6302) knots 0 0 0 1 2 2 2
  spline S54 degree 2 poles (67.7108, 23.6302) (67.8186, 23.7749) (68.1617, 23.9167) (68.4085, 23.9167) knots 0 0 0 1 2 2 2
  line L71 (68.4085, 23.9167) -> (70.2039, 23.9167)
  line L72 (70.2039, 23.9167) -> (70.2039, 23.4742)
  line L73 (70.2039, 23.4742) -> (69.9259, 23.4742)
  line L74 (69.5572, 23.4742) -> (68.8283, 23.4742)
  spline S55 degree 2 poles (68.8283, 23.4742) (68.8425, 23.3154) (68.8907, 22.8361) (68.9361, 22.6857) knots 0 0 0 1 2 2 2
  spline S56 degree 2 poles (68.9361, 22.6857) (68.9899, 22.5099) (69.214, 22.2801) (69.4126, 22.2801) knots 0 0 0 1 2 2 2
  spline S57 degree 2 poles (69.4126, 22.2801) (69.6395, 22.2801) (69.8692, 22.5354) (69.8692, 22.7793) knots 0 0 0 1 2 2 2
  spline S58 degree 2 poles (69.8692, 22.7793) (69.8692, 22.9864) (69.6905, 23.3267) (69.5572, 23.4742) knots 0 0 0 1 2 2 2
  spline S59 degree 2 poles (70.2663, 25.2469) (70.2663, 24.9831) (70.1245, 24.5265) (70.0451, 24.3762) knots 0 0 0 1 2 2 2
  line L75 (70.0451, 24.3762) -> (69.5487, 24.3762)
  line L76 (69.5487, 24.3762) -> (69.5487, 24.3989)
  spline S60 degree 2 poles (69.5487, 24.3989) (69.5941, 24.4556) (69.7019, 24.6087) (69.7614, 24.7364) knots 0 0 0 1 2 2 2
  spline S61 degree 2 poles (69.7614, 24.7364) (69.8153, 24.847) (69.8947, 25.1193) (69.8947, 25.2639) knots 0 0 0 1 2 2 2
  spline S62 degree 2 poles (69.8947, 25.2639) (69.8947, 25.3689) (69.8465, 25.61) (69.8068, 25.6667) knots 0 0 0 1 2 2 2
  spline S63 degree 2 poles (69.8068, 25.6667) (69.7529, 25.7489) (69.631, 25.8227) (69.5062, 25.8227) knots 0 0 0 1 2 2 2
  spline S64 degree 2 poles (69.5062, 25.8227) (69.3502, 25.8227) (69.1885, 25.6525) (69.1346, 25.4341) knots 0 0 0 1 2 2 2
  spline S65 degree 2 poles (69.1346, 25.4341) (69.1147, 25.349) (69.058, 25.0767) (69.0268, 24.9605) knots 0 0 0 1 2 2 2
  spline S66 degree 2 poles (69.0268, 24.9605) (68.9389, 24.6598) (68.5758, 24.3875) (68.3177, 24.3875) knots 0 0 0 1 2 2 2
  spline S67 degree 2 poles (68.3177, 24.3875) (67.9604, 24.3875) (67.5151, 24.9236) (67.5151, 25.366) knots 0 0 0 1 2 2 2
  spline S68 degree 2 poles (67.5151, 25.366) (67.5151, 25.5844) (67.6229, 26.0269) (67.7051, 26.1772) knots 0 0 0 1 2 2 2
  line L77 (67.7051, 26.1772) -> (68.1788, 26.1772)
  line L78 (68.1788, 26.1772) -> (68.1788, 26.1545)
  spline S69 degree 2 poles (68.1788, 26.1545) (68.0426, 25.9844) (67.8866, 25.5703) (67.8866, 25.3575) knots 0 0 0 1 2 2 2
  spline S70 degree 2 poles (67.8866, 25.3575) (67.8866, 25.1391) (68.071, 24.8385) (68.2553, 24.8385) knots 0 0 0 1 2 2 2
  spline S71 degree 2 poles (68.2553, 24.8385) (68.4227, 24.8385) (68.5844, 25.0172) (68.6354, 25.2157) knots 0 0 0 1 2 2 2
  spline S72 degree 2 poles (68.6354, 25.2157) (68.6609, 25.3122) (68.712, 25.5561) (68.7432, 25.6894) knots 0 0 0 1 2 2 2
  spline S73 degree 2 poles (68.7432, 25.6894) (68.8169, 25.9787) (69.1545, 26.2737) (69.4466, 26.2737) knots 0 0 0 1 2 2 2
  spline S74 degree 2 poles (69.4466, 26.2737) (69.6168, 26.2737) (69.9174, 26.1404) (70.028, 26.0099) knots 0 0 0 1 2 2 2
  spline S75 degree 2 poles (70.028, 26.0099) (70.1443, 25.8709) (70.2663, 25.5164) (70.2663, 25.2469) knots 0 0 0 1 2 2 2
  line L79 (67.5775, 28.7469) -> (71.1711, 27.3344)
  line L80 (71.1711, 27.3344) -> (71.1711, 26.8608)
  line L81 (71.1711, 26.8608) -> (70.0763, 27.3316)
  line L82 (70.0763, 27.3316) -> (67.5775, 26.3786)
  line L83 (67.5775, 26.3786) -> (67.5775, 26.8551)
  line L84 (67.5775, 26.8551) -> (69.5232, 27.5727)
  line L85 (69.5232, 27.5727) -> (67.5775, 28.2874)
  line L86 (67.5775, 28.2874) -> (67.5775, 28.7469)
  spline S76 degree 2 poles (70.2635, 30.1254) (70.2635, 29.8531) (70.0961, 29.4021) (69.9259, 29.2404) knots 0 0 0 1 2 2 2
  spline S77 degree 2 poles (69.9259, 29.2404) (69.7586, 29.0788) (69.2424, 28.9001) (68.8964, 28.9001) knots 0 0 0 1 2 2 2
  spline S78 degree 2 poles (68.8964, 28.9001) (68.5503, 28.9001) (68.0455, 29.0844) (67.8753, 29.2404) knots 0 0 0 1 2 2 2
  spline S79 degree 2 poles (67.8753, 29.2404) (67.7023, 29.3964) (67.5179, 29.8587) (67.5179, 30.1254) knots 0 0 0 1 2 2 2
  spline S80 degree 2 poles (67.5179, 30.1254) (67.5179, 30.3409) (67.6399, 30.7437) (67.7193, 30.8997) knots 0 0 0 1 2 2 2
  line L87 (67.7193, 30.8997) -> (68.2156, 30.8997)
  line L88 (68.2156, 30.8997) -> (68.2156, 30.8741)
  spline S81 degree 2 poles (68.2156, 30.8741) (68.1759, 30.8259) (68.0738, 30.6784) (68.0199, 30.5735) knots 0 0 0 1 2 2 2
  spline S82 degree 2 poles (68.0199, 30.5735) (67.9746, 30.4799) (67.9036, 30.2303) (67.9036, 30.1169) knots 0 0 0 1 2 2 2
  spline S83 degree 2 poles (67.9036, 30.1169) (67.9036, 29.7737) (68.4227, 29.3567) (68.8964, 29.3567) knots 0 0 0 1 2 2 2
  spline S84 degree 2 poles (68.8964, 29.3567) (69.3587, 29.3567) (69.8777, 29.7595) (69.8777, 30.1169) knots 0 0 0 1 2 2 2
  spline S85 degree 2 poles (69.8777, 30.1169) (69.8777, 30.3324) (69.699, 30.7238) (69.56, 30.8741) knots 0 0 0 1 2 2 2
  line L89 (69.56, 30.8741) -> (69.56, 30.8997)
  line L90 (69.56, 30.8997) -> (70.0564, 30.8997)
  spline S86 degree 2 poles (70.0564, 30.8997) (70.0876, 30.8344) (70.1755, 30.6359) (70.1954, 30.5565) knots 0 0 0 1 2 2 2
  spline S87 degree 2 poles (70.1954, 30.5565) (70.2294, 30.443) (70.2635, 30.2643) (70.2635, 30.1254) knots 0 0 0 1 2 2 2
  line L91 (75.9665, 11.8454) -> (75.9665, 9.8174)
  line L92 (75.9665, 9.8174) -> (72.4665, 9.8174)
  line L93 (72.4665, 9.8174) -> (72.4665, 10.2826)
  line L94 (72.4665, 10.2826) -> (75.5524, 10.2826)
  line L95 (75.5524, 10.2826) -> (75.5524, 11.8454)
  line L96 (75.5524, 11.8454) -> (75.9665, 11.8454)
  spline S88 degree 2 poles (75.6886, 13.6408) (75.7283, 13.5869) (75.8701, 13.4053) (75.9127, 13.3203) knots 0 0 0 1 2 2 2
  spline S89 degree 2 poles (75.9127, 13.3203) (75.9751, 13.204) (76.0403, 12.9856) (76.0403, 12.787) knots 0 0 0 1 2 2 2
  spline S90 degree 2 poles (76.0403, 12.787) (76.0403, 12.6254) (75.9183, 12.3332) (75.8077, 12.2226) knots 0 0 0 1 2 2 2
  spline S91 degree 2 poles (75.8077, 12.2226) (75.6999, 12.1177) (75.3823, 11.99) (75.2064, 11.99) knots 0 0 0 1 2 2 2
  spline S92 degree 2 poles (75.2064, 11.99) (74.9341, 11.99) (74.5484, 12.2198) (74.4378, 12.4694) knots 0 0 0 1 2 2 2
  spline S93 degree 2 poles (74.4378, 12.4694) (74.3357, 12.6906) (74.2591, 13.2919) (74.2392, 13.6408) knots 0 0 0 1 2 2 2
  line L97 (74.2392, 13.6408) -> (74.1541, 13.6408)
  spline S94 degree 2 poles (74.1541, 13.6408) (74.001, 13.6408) (73.811, 13.5472) (73.7571, 13.4621) knots 0 0 0 1 2 2 2
  spline S95 degree 2 poles (73.7571, 13.4621) (73.7032, 13.377) (73.6691, 13.1331) (73.6691, 13.0026) knots 0 0 0 1 2 2 2
  spline S96 degree 2 poles (73.6691, 13.0026) (73.6691, 12.8494) (73.7599, 12.4353) (73.8478, 12.2283) knots 0 0 0 1 2 2 2
  line L98 (73.8478, 12.2283) -> (73.8478, 12.2028)
  line L99 (73.8478, 12.2028) -> (73.3969, 12.2028)
  spline S97 degree 2 poles (73.3969, 12.2028) (73.3628, 12.3247) (73.2777, 12.7814) (73.2777, 13.0054) knots 0 0 0 1 2 2 2
  spline S98 degree 2 poles (73.2777, 13.0054) (73.2777, 13.2777) (73.3628, 13.6493) (73.4734, 13.7968) knots 0 0 0 1 2 2 2
  spline S99 degree 2 poles (73.4734, 13.7968) (73.5812, 13.9414) (73.9244, 14.0832) (74.1712, 14.0832) knots 0 0 0 1 2 2 2
  line L100 (74.1712, 14.0832) -> (75.9665, 14.0832)
  line L101 (75.9665, 14.0832) -> (75.9665, 13.6408)
  line L102 (75.9665, 13.6408) -> (75.6886, 13.6408)
  line L103 (75.3199, 13.6408) -> (74.5909, 13.6408)
  spline S100 degree 2 poles (74.5909, 13.6408) (74.6051, 13.4819) (74.6533, 13.0026) (74.6987, 12.8523) knots 0 0 0 1 2 2 2
  spline S101 degree 2 poles (74.6987, 12.8523) (74.7526, 12.6764) (74.9767, 12.4467) (75.1752, 12.4467) knots 0 0 0 1 2 2 2
  spline S102 degree 2 poles (75.1752, 12.4467) (75.4021, 12.4467) (75.6319, 12.7019) (75.6319, 12.9459) knots 0 0 0 1 2 2 2
  spline S103 degree 2 poles (75.6319, 12.9459) (75.6319, 13.1529) (75.4532, 13.4933) (75.3199, 13.6408) knots 0 0 0 1 2 2 2
  spline S104 degree 2 poles (74.6108, 16.9053) (75.2546, 16.9053) (76.0403, 16.2814) (76.0403, 15.8105) knots 0 0 0 1 2 2 2
  spline S105 degree 2 poles (76.0403, 15.8105) (76.0403, 15.5978) (75.9353, 15.2943) (75.8446, 15.1468) knots 0 0 0 1 2 2 2
  line L104 (75.8446, 15.1468) -> (75.9665, 15.1185)
  line L105 (75.9665, 15.1185) -> (75.9665, 14.7044)
  line L106 (75.9665, 14.7044) -> (72.3105, 14.7044)
  line L107 (72.3105, 14.7044) -> (72.3105, 15.1468)
  line L108 (72.3105, 15.1468) -> (73.6152, 15.1468)
  spline S106 degree 2 poles (73.6152, 15.1468) (73.4649, 15.3142) (73.2664, 15.7028) (73.2664, 15.9495) knots 0 0 0 1 2 2 2
  spline S107 degree 2 poles (73.2664, 15.9495) (73.2664, 16.3948) (73.9783, 16.9053) (74.6108, 16.9053) knots 0 0 0 1 2 2 2
  spline S108 degree 2 poles (74.6448, 16.4487) (74.174, 16.4487) (73.6862, 16.1622) (73.6862, 15.8446) knots 0 0 0 1 2 2 2
  spline S109 degree 2 poles (73.6862, 15.8446) (73.6862, 15.6659) (73.8563, 15.2972) (73.9868, 15.1468) knots 0 0 0 1 2 2 2
  line L109 (73.9868, 15.1468) -> (75.4929, 15.1468)
  spline S110 degree 2 poles (75.4929, 15.1468) (75.5751, 15.3142) (75.6432, 15.5723) (75.6432, 15.7254) knots 0 0 0 1 2 2 2
  spline S111 degree 2 poles (75.6432, 15.7254) (75.6432, 16.063) (75.1639, 16.4487) (74.6448, 16.4487) knots 0 0 0 1 2 2 2
  point P0 (0, 0)
  constraints: 4 other
emboss "Gravure1" sketch "Esquisse9" operation cut depth 1 direction (0, 0, 1)
sketch "Esquisse10" plane through (0, 0, -2) normal (0, 0, -1) x (-1, 0, 0)
  line L0 (75.5524, 11.8454) -> (75.9665, 11.8454) projected
  line L1 (75.9665, 11.8454) -> (75.9665, 9.8174) projected
  line L2 (75.9665, 9.8174) -> (72.4665, 9.8174) projected
  line L3 (72.4665, 9.8174) -> (72.4665, 10.2826) projected
  line L4 (72.4665, 10.2826) -> (75.5524, 10.2826) projected
  line L5 (75.5524, 10.2826) -> (75.5524, 11.8454) projected
  line L6 (66.7039, 10.2826) -> (68.0767, 10.2826) projected
  line L7 (68.0767, 10.2826) -> (68.0767, 11.8936) projected
  line L8 (68.0767, 11.8936) -> (66.7039, 11.8936) projected
  line L9 (66.7039, 11.8936) -> (66.7039, 12.3587) projected
  line L10 (66.7039, 12.3587) -> (70.2039, 12.3587) projected
  line L11 (70.2039, 12.3587) -> (70.2039, 11.8936) projected
  line L12 (70.2039, 11.8936) -> (68.4908, 11.8936) projected
  line L13 (68.4908, 11.8936) -> (68.4908, 10.2826) projected
  line L14 (68.4908, 10.2826) -> (70.2039, 10.2826) projected
  line L15 (70.2039, 10.2826) -> (70.2039, 9.8174) projected
  line L16 (70.2039, 9.8174) -> (66.7039, 9.8174) projected
  line L17 (66.7039, 9.8174) -> (66.7039, 10.2826) projected
  line L18 (27.5395, 14.7544) -> (28.1723, 14.7544) projected
  line L19 (28.1723, 14.7544) -> (28.1723, 9.2574) projected
  line L20 (28.1723, 9.2574) -> (29.2548, 9.2574) projected
  line L21 (29.2548, 9.2574) -> (29.2548, 8.6346) projected
  line L22 (29.2548, 8.6346) -> (26.279, 8.6346) projected
  line L23 (26.279, 8.6346) -> (26.279, 9.2574) projected
  line L24 (26.279, 9.2574) -> (27.3863, 9.2574) projected
  line L25 (27.3863, 9.2574) -> (27.3863, 13.3455) projected
  line L26 (27.3863, 13.3455) -> (26.279, 13.3455) projected
  line L27 (26.279, 13.3455) -> (26.279, 13.9041) projected
  line L28 (67.6824, 19.8267) -> (66.5479, 19.8267) projected
  line L29 (66.5479, 19.8267) -> (66.5479, 20.2692) projected
  line L30 (66.5479, 20.2692) -> (70.2039, 20.2692) projected
  line L31 (70.2039, 20.2692) -> (70.2039, 19.8267) projected
  line L32 (70.2039, 19.8267) -> (69.9373, 19.8267) projected
  line L33 (22.8731, 9.6677) -> (24.5637, 14.7346) projected
  line L34 (24.5637, 14.7346) -> (25.3892, 14.7346) projected
  line L35 (25.3892, 14.7346) -> (23.2883, 8.6346) projected
  line L36 (23.2883, 8.6346) -> (22.4134, 8.6346) projected
  line L37 (22.4134, 8.6346) -> (20.3125, 14.7346) projected
  line L38 (20.3125, 14.7346) -> (21.1825, 14.7346) projected
  line L39 (21.1825, 14.7346) -> (22.8731, 9.6677) projected
  line L40 (67.5775, 21.3612) -> (70.2039, 21.3612) projected
  line L41 (70.2039, 21.3612) -> (70.2039, 20.9187) projected
  line L42 (70.2039, 20.9187) -> (67.5775, 20.9187) projected
  line L43 (67.5775, 20.9187) -> (67.5775, 21.3612) projected
  line L44 (31.6869, 8.6346) -> (30.7082, 8.6346) projected
  line L45 (30.7082, 8.6346) -> (30.7082, 9.8012) projected
  line L46 (30.7082, 9.8012) -> (31.6869, 9.8012) projected
  line L47 (31.6869, 9.8012) -> (31.6869, 8.6346) projected
  line L48 (68.0852, 22.0617) -> (68.0852, 22.0362) projected
  line L49 (68.0852, 22.0362) -> (67.6342, 22.0362) projected
  line L50 (68.4085, 23.9167) -> (70.2039, 23.9167) projected
  line L51 (70.2039, 23.9167) -> (70.2039, 23.4742) projected
  line L52 (70.2039, 23.4742) -> (69.9259, 23.4742) projected
  line L53 (68.4766, 23.4742) -> (68.3915, 23.4742) projected
  line L54 (69.56, 15.0447) -> (69.56, 15.0703) projected
  line L55 (69.56, 15.0703) -> (70.0422, 15.0703) projected
  line L56 (68.695, 15.1185) -> (68.9361, 15.1185) projected
  line L57 (68.9361, 15.1185) -> (68.9361, 13.3004) projected
  line L58 (67.7051, 26.1772) -> (68.1788, 26.1772) projected
  line L59 (68.1788, 26.1772) -> (68.1788, 26.1545) projected
  line L60 (70.0451, 24.3762) -> (69.5487, 24.3762) projected
  line L61 (69.5487, 24.3762) -> (69.5487, 24.3989) projected
  line L62 (69.5402, 17.1663) -> (67.5775, 17.1663) projected
  line L63 (67.5775, 17.1663) -> (67.5775, 17.6087) projected
  line L64 (67.5775, 17.6087) -> (70.2039, 17.6087) projected
  line L65 (70.2039, 17.6087) -> (70.2039, 17.1663) projected
  line L66 (70.2039, 17.1663) -> (69.9146, 17.1663) projected
  line L67 (69.2821, 15.5468) -> (67.5775, 15.5468) projected
  line L68 (67.5775, 15.5468) -> (67.5775, 15.9892) projected
  line L69 (67.5775, 15.9892) -> (69.075, 15.9892) projected
  line L70 (69.56, 30.8741) -> (69.56, 30.8997) projected
  line L71 (69.56, 30.8997) -> (70.0564, 30.8997) projected
  line L72 (67.7193, 30.8997) -> (68.2156, 30.8997) projected
  line L73 (68.2156, 30.8997) -> (68.2156, 30.8741) projected
  line L74 (67.1407, 21.3924) -> (67.1407, 20.8904) projected
  line L75 (67.1407, 20.8904) -> (66.6812, 20.8904) projected
  line L76 (66.6812, 20.8904) -> (66.6812, 21.3924) projected
  line L77 (66.6812, 21.3924) -> (67.1407, 21.3924) projected
  line L78 (73.8478, 12.2283) -> (73.8478, 12.2028) projected
  line L79 (73.8478, 12.2028) -> (73.3969, 12.2028) projected
  line L80 (74.1712, 14.0832) -> (75.9665, 14.0832) projected
  line L81 (75.9665, 14.0832) -> (75.9665, 13.6408) projected
  line L82 (75.9665, 13.6408) -> (75.6886, 13.6408) projected
  line L83 (74.2392, 13.6408) -> (74.1541, 13.6408) projected
  line L84 (69.5232, 27.5727) -> (67.5775, 28.2874) projected
  line L85 (67.5775, 28.2874) -> (67.5775, 28.7469) projected
  line L86 (67.5775, 28.7469) -> (71.1711, 27.3344) projected
  line L87 (71.1711, 27.3344) -> (71.1711, 26.8608) projected
  line L88 (71.1711, 26.8608) -> (70.0763, 27.3316) projected
  line L89 (70.0763, 27.3316) -> (67.5775, 26.3786) projected
  line L90 (67.5775, 26.3786) -> (67.5775, 26.8551) projected
  line L91 (67.5775, 26.8551) -> (69.5232, 27.5727) projected
  line L92 (72.3105, 14.7044) -> (72.3105, 15.1468) projected
  line L93 (72.3105, 15.1468) -> (73.6152, 15.1468) projected
  line L94 (75.8446, 15.1468) -> (75.9665, 15.1185) projected
  line L95 (75.9665, 15.1185) -> (75.9665, 14.7044) projected
  line L96 (75.9665, 14.7044) -> (72.3105, 14.7044) projected
  line L97 (9, 16) -> (6, 16) projected
  line L98 (6, 16) -> (6, 19) projected
  line L99 (6, 19) -> (9, 19) projected
  line L100 (9, 19) -> (9, 16) projected
  circle A0 centre (60, 33.25) radius 1 projected
  circle A1 centre (71.5, 55) radius 1 projected
  circle A2 centre (65, 55) radius 1 projected
  circle A3 centre (40, 26.75) radius 1 projected
  circle A4 centre (28.5, 5) radius 1 projected
  circle A5 centre (35, 5) radius 1 projected
  line L101 (14, 15) -> (14, 20) projected
  line L102 (14, 20) -> (19, 20) projected
  line L103 (19, 20) -> (19, 15) projected
  line L104 (19, 15) -> (14, 15) projected
  line L105 (9, 41) -> (6, 41) projected
  line L106 (6, 41) -> (6, 44) projected
  line L107 (6, 44) -> (9, 44) projected
  line L108 (9, 44) -> (9, 41) projected
  line L109 (19, 45) -> (19, 40) projected
  line L110 (19, 40) -> (14, 40) projected
  line L111 (14, 40) -> (14, 45) projected
  line L112 (14, 45) -> (19, 45) projected
  circle A6 centre (28.5, 55) radius 1 projected
  circle A7 centre (35, 55) radius 1 projected
  circle A8 centre (40, 33.25) radius 1 projected
  line L113 (61.2, 45.5) -> (61.1821, 45.5) projected
  line L114 (61.1821, 45.5) -> (61.1821, 42) projected
  line L115 (61.1821, 42) -> (38.8, 42) projected
  line L116 (38.8, 42) -> (38.8, 60) projected
  line L117 (38.8, 60) -> (23, 60) projected
  arc A9 (23, 60) -> (19, 56) centre (23, 56) ccw projected
  line L118 (19, 56) -> (19, 48) projected
  line L119 (19, 48) -> (3.3524, 48) projected
  arc A10 (3.3524, 48) -> (3.3524, 12) centre (50, 30) ccw projected
  line L120 (3.3524, 12) -> (19, 12) projected
  line L121 (19, 12) -> (19, 4) projected
  arc A11 (19, 4) -> (23, 0) centre (23, 4) ccw projected
  line L122 (23, 0) -> (38.8, 0) projected
  line L123 (38.8, 0) -> (38.8, 18) projected
  line L124 (38.8, 18) -> (61.1821, 18) projected
  line L125 (61.1821, 18) -> (61.1821, 14.5) projected
  line L126 (61.1821, 14.5) -> (61.2, 14.5) projected
  line L127 (61.2, 14.5) -> (61.2, 0) projected
  line L128 (61.2, 0) -> (77, 0) projected
  arc A12 (77, 0) -> (81, 4) centre (77, 4) ccw projected
  line L129 (81, 4) -> (81, 12) projected
  line L130 (81, 12) -> (96.6476, 12) projected
  arc A13 (96.6476, 12) -> (96.6476, 48) centre (50, 30) ccw projected
  line L131 (96.6476, 48) -> (81, 48) projected
  line L132 (81, 48) -> (81, 56) projected
  arc A14 (81, 56) -> (77, 60) centre (77, 56) ccw projected
  line L133 (77, 60) -> (61.2, 60) projected
  line L134 (61.2, 60) -> (61.2, 45.5) projected
  circle A15 centre (60, 26.75) radius 1 projected
  circle A16 centre (71.5, 5) radius 1 projected
  circle A17 centre (65, 5) radius 1 projected
  line L135 (81, 20) -> (86, 20) projected
  line L136 (86, 20) -> (86, 15) projected
  line L137 (86, 15) -> (81, 15) projected
  line L138 (81, 15) -> (81, 20) projected
  line L139 (91, 19) -> (94, 19) projected
  line L140 (94, 19) -> (94, 16) projected
  line L141 (94, 16) -> (91, 16) projected
  line L142 (91, 16) -> (91, 19) projected
  line L143 (86, 45) -> (86, 40) projected
  line L144 (86, 40) -> (81, 40) projected
  line L145 (81, 40) -> (81, 45) projected
  line L146 (81, 45) -> (86, 45) projected
  line L147 (91, 44) -> (94, 44) projected
  line L148 (94, 44) -> (94, 41) projected
  line L149 (94, 41) -> (91, 41) projected
  line L150 (91, 41) -> (91, 44) projected
  circle A18 centre (7.5, 42.5) radius 1.5
  circle A19 centre (7.5, 17.5) radius 1.5
  circle A20 centre (92.5, 42.5) radius 1.5
  circle A21 centre (92.5, 17.5) radius 1.5
  circle A22 centre (16.5, 17.5) radius 2.5
  circle A23 centre (16.5, 42.5) radius 2.5
  circle A24 centre (83.5, 17.5) radius 2.5
  circle A25 centre (83.5, 42.5) radius 2.5
  constraints: 24 tangent, 8 centre point, 84 other